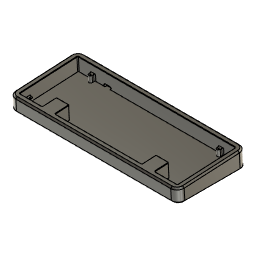
Vault 35 WKL MFR2 (Autodesk Fusion 360 design; units mm, degrees)
Autodesk Fusion 360 part; units mm, degrees
sketch "Outline Sketch" plane through (0, 0, 0) normal (0, 0, 1) x (1, 0, 0)
  line L0 (12.0219, -2.3777) -> (12.0219, 74.0723) construction
  line L1 (12.0219, 74.0723) -> (221.8219, 74.0723) construction
  line L2 (221.8219, 74.0723) -> (221.8219, -2.3777) construction
  line L3 (221.8219, -2.3777) -> (192.9969, -2.3777) construction
  line L4 (192.9969, -2.3777) -> (192.9969, 16.6723) construction
  line L5 (192.9969, 16.6723) -> (174.1969, 16.6723) construction
  line L6 (174.1969, 16.6723) -> (174.1969, -2.3777) construction
  line L7 (174.1969, -2.3777) -> (59.6469, -2.3777) construction
  line L8 (59.6469, -2.3777) -> (59.6469, 16.6723) construction
  line L9 (59.6469, 16.6723) -> (40.8469, 16.6723) construction
  line L10 (40.8469, 16.6723) -> (40.8469, -2.3777) construction
  line L11 (40.8469, -2.3777) -> (12.0219, -2.3777) construction
  line L12 (222.5719, -3.1277) -> (192.2469, -3.1277)
  line L13 (192.2469, -3.1277) -> (192.2469, 15.9223)
  line L14 (192.2469, 15.9223) -> (174.9469, 15.9223)
  line L15 (174.9469, 15.9223) -> (174.9469, -3.1277)
  line L16 (174.9469, -3.1277) -> (58.8969, -3.1277)
  line L17 (58.8969, -3.1277) -> (58.8969, 15.9223)
  line L18 (58.8969, 15.9223) -> (41.5969, 15.9223)
  line L19 (41.5969, 15.9223) -> (41.5969, -3.1277)
  line L20 (41.5969, -3.1277) -> (11.2719, -3.1277)
  line L21 (11.2719, -3.1277) -> (11.2719, 74.8223)
  line L22 (11.2719, 74.8223) -> (222.5719, 74.8223)
  line L23 (222.5719, 74.8223) -> (222.5719, -3.1277)
  line L24 (229.5719, -10.1277) -> (185.2469, -10.1277)
  line L25 (185.2469, -10.1277) -> (185.2469, 8.9223)
  line L26 (185.2469, 8.9223) -> (181.9469, 8.9223)
  line L27 (181.9469, 8.9223) -> (181.9469, -10.1277)
  line L28 (181.9469, -10.1277) -> (51.8969, -10.1277)
  line L29 (51.8969, -10.1277) -> (51.8969, 8.9223)
  line L30 (51.8969, 8.9223) -> (48.5969, 8.9223)
  line L31 (48.5969, 8.9223) -> (48.5969, -10.1277)
  line L32 (48.5969, -10.1277) -> (4.2719, -10.1277)
  line L33 (4.2719, -10.1277) -> (4.2719, 81.8223)
  line L34 (4.2719, 81.8223) -> (229.5719, 81.8223)
  line L35 (229.5719, 81.8223) -> (229.5719, -10.1277)
  line L36 (48.5969, -10.1277) -> (51.8969, -10.1277)
  line L37 (181.9469, -10.1277) -> (185.2469, -10.1277)
  dimension "d1" = 209.8
  dimension "d2" = 76.45
  dimension "d3" = 28.825
  dimension "d4" = 28.825
  dimension "d6" = 18.8
  dimension "d7" = 18.8
  dimension "d9" = 19.05
  dimension "d10" = 19.05
  dimension "d11" = 19.05
  dimension "d12" = 76.45
  dimension "d13" = 114.55
  dimension "d14" = -0.75
  dimension "d15" = -7.75
  constraint vertical L0
  constraint perpendicular L0 L1
  constraint perpendicular L1 L2
  constraint perpendicular L2 L3
  constraint perpendicular L3 L4
  constraint perpendicular L4 L5
  constraint perpendicular L5 L6
  constraint perpendicular L6 L7
  constraint perpendicular L7 L8
  constraint perpendicular L8 L9
  constraint perpendicular L9 L10
  constraint perpendicular L0 L11
  measures "d1" distance of L0 L2
  measures "d2" distance of L0.start L0.end
  measures "d3" distance of L0.start L10.end
  measures "d4" distance of L2.end L3.end
  measures "d6" distance of L8 L10
  measures "d7" distance of L4 L6
  measures "d9" distance of L9 L11
  measures "d10" distance of L3 L5
  measures "d11" distance of L7 L9
  measures "d12" distance of L1.end L2.end
  measures "d13" distance of L6 L8
extrude "Extrude1" add sketch "Outline Sketch" along normal blind 18.06
sketch "Angle Sketch" plane through (229.5719, 0, 0) normal (1, 0, 0) x (0, 1, 0)
  line L0 (-10.1277, 0) -> (81.8223, 0)
  line L1 (81.8223, 0) -> (81.8223, 18.06)
  line L2 (81.8223, 18.06) -> (-10.1277, 18.06)
  line L3 (-10.1277, 18.06) -> (-10.1277, 0)
  line L4 (-10.1277, 18.06) -> (-10.1277, -0.215)
  line L5 (-10.1277, -0.215) -> (89.7352, -5.4486)
  line L6 (-10.1277, -0.215) -> (89.8723, -0.215) construction
  dimension "d18" = 18.275
  dimension "d19" = 100
  dimension "d20" = 3
  constraint coincident L2.end L3.start
  constraint perpendicular L0 L4
  constraint horizontal L6
  measures "d18" distance of L2.end L4.end
  measures "d19" distance of L4.end L5.end
  measures "d20" angle of L5 L6
ref_plane "WorkPlane1" through (229.5719, 39.8037, -2.8318) normal (0, -0.052336, -0.99863) x (0, 0.99863, -0.052336)
sketch "Bottom Sketch for Angle" plane through (0, 0, 0) normal (0, 0, -1) x (1, 0, 0)
  line L0 (222.5719, -74.8223) -> (11.2719, -74.8223)
  line L1 (11.2719, -74.8223) -> (11.2719, 3.1277)
  line L2 (11.2719, 3.1277) -> (41.5969, 3.1277)
  line L3 (41.5969, 3.1277) -> (41.5969, -15.9223)
  line L4 (41.5969, -15.9223) -> (58.8969, -15.9223)
  line L5 (58.8969, -15.9223) -> (58.8969, 3.1277)
  line L6 (58.8969, 3.1277) -> (174.9469, 3.1277)
  line L7 (174.9469, 3.1277) -> (174.9469, -15.9223)
  line L8 (174.9469, -15.9223) -> (192.2469, -15.9223)
  line L9 (192.2469, -15.9223) -> (192.2469, 3.1277)
  line L10 (192.2469, 3.1277) -> (222.5719, 3.1277)
  line L11 (222.5719, 3.1277) -> (222.5719, -74.8223)
  line L12 (229.5719, 10.1277) -> (4.2719, 10.1277)
  line L13 (4.2719, 10.1277) -> (4.2719, -81.8223)
  line L14 (4.2719, -81.8223) -> (229.5719, -81.8223)
  line L15 (229.5719, -81.8223) -> (229.5719, 10.1277)
  line L16 (229.5719, -81.8223) -> (4.2719, -81.8223)
  line L17 (4.2719, -81.8223) -> (4.2719, 10.1277)
  line L18 (4.2719, 10.1277) -> (229.5719, 10.1277)
  line L19 (229.5719, 10.1277) -> (229.5719, -81.8223)
  constraint horizontal L16
  constraint vertical L17
  constraint horizontal L18
  constraint vertical L19
  constraint coincident L12.end L13.start
  constraint coincident L14.end L15.start
extrude "Extrude2" add sketch "Bottom Sketch for Angle" along normal up to surface contours L0 L1 L2 L3 L4 L5 L6 L7 L8 L9 L10 L11 | L12 L13 L14 L15 L16 L17 L18 L19 end surface through (229.5719, 39.8037, -2.8318) normal (0, -0.052336, -0.99863) offset 0
sketch "USB C Hole Internal Sketch" plane through (0, 74.8223, 0) normal (0, -1, 0) x (1, 0, 0)
  line L0 (11.2719, 0) -> (222.5719, 0)
  line L1 (222.5719, 0) -> (222.5719, 18.06)
  line L2 (222.5719, 18.06) -> (11.2719, 18.06)
  line L3 (11.2719, 18.06) -> (11.2719, 0)
  line L4 (11.2719, 0) -> (50.2469, 0) construction
  line L5 (50.2469, 0) -> (50.2469, 1.83) construction
  line L6 (54.9719, 3.66) -> (45.5219, 3.66)
  line L7 (45.5219, 3.66) -> (45.5219, 0)
  line L8 (45.5219, 0) -> (54.9719, 0)
  line L9 (54.9719, 0) -> (54.9719, 3.66)
  line L10 (54.9719, 3.66) -> (45.5219, 0) construction
  line L11 (45.5219, 3.66) -> (54.9719, 0) construction
  point P0 (50.2469, 1.83)
  dimension "d62" = 38.975
  dimension "d63" = 1.83
  dimension "d64" = 9.45
  dimension "d65" = 3.66
  constraint coincident L0.start L3.end
  constraint perpendicular L3 L4
  constraint perpendicular L4 L5
  constraint horizontal L6
  constraint perpendicular L6 L7
  constraint parallel L6 L8
  constraint parallel L7 L9
  constraint coincident L10 P0
  constraint coincident L11 P0
  constraint coincident P0 L5.end
  measures "d62" distance of L0.start L4.end
  measures "d63" distance of L4.end P0
  measures "d64" distance of L7.end L8.end
  measures "d65" distance of L6.end L7.end
extrude "Extrude5" cut sketch "USB C Hole Internal Sketch" against normal through all contours L0 L6 L7 L8 L9
fillet "Fillet3" radius 1.55 4 edges at (45.5219, 78.3223, 0) (54.9719, 78.3223, 0) (54.9719, 78.3223, 3.66) (45.5219, 78.3223, 3.66)
sketch "USB C Hole External Sketch" plane through (0, 81.8223, 0) normal (0, 1, 0) x (-1, 0, 0)
  line L0 (-47.0719, 0) -> (-53.4219, 0)
  arc A0 (-54.9719, 1.55) -> (-53.4219, 0) centre (-53.4219, 1.55) ccw
  line L1 (-54.9719, 1.55) -> (-54.9719, 2.11)
  arc A1 (-53.4219, 3.66) -> (-54.9719, 2.11) centre (-53.4219, 2.11) ccw
  line L2 (-53.4219, 3.66) -> (-47.0719, 3.66)
  arc A2 (-45.5219, 2.11) -> (-47.0719, 3.66) centre (-47.0719, 2.11) ccw
  line L3 (-45.5219, 2.11) -> (-45.5219, 1.55)
  arc A3 (-47.0719, 0) -> (-45.5219, 1.55) centre (-47.0719, 1.55) ccw
  line L4 (-4.2719, -5.0339) -> (-4.2719, 18.06)
  line L5 (-4.2719, 18.06) -> (-229.5719, 18.06)
  line L6 (-229.5719, 18.06) -> (-229.5719, -5.0339)
  line L7 (-229.5719, -5.0339) -> (-4.2719, -5.0339)
  line L8 (-43.2719, 5.91) -> (-57.2219, 5.91)
  line L9 (-57.2219, 5.91) -> (-57.2219, -2.25)
  line L10 (-57.2219, -2.25) -> (-43.2719, -2.25)
  line L11 (-43.2719, -2.25) -> (-43.2719, 5.91)
  line L12 (-43.2719, 5.91) -> (-57.2219, -2.25) construction
  line L13 (-57.2219, 5.91) -> (-43.2719, -2.25) construction
  point P0 (-50.2469, 1.83)
  point P1 (-50.2469, 1.83)
  dimension "d69" = 13.95
  dimension "d70" = 8.16
  dimension "d71" = 4.08
  dimension "d72" = 6.975
  constraint horizontal L8
  constraint perpendicular L8 L9
  constraint parallel L8 L10
  constraint parallel L9 L11
  constraint coincident L12 P1
  constraint coincident L13 P1
  measures "d69" distance of L9.end L10.end
  measures "d70" distance of L8.end L9.end
  measures "d71" distance of L8 P1
  measures "d72" distance of L9 P1
extrude "Extrude6" cut sketch "USB C Hole External Sketch" against normal blind 4.549 contours L8 L9 L10 L11
fillet "Fillet4" radius 3.8 4 edges at (57.2219, 79.5478, -2.25) (57.2219, 79.5478, 5.91) (43.2719, 79.5478, -2.25) (43.2719, 79.5478, 5.91)
chamfer "Chamfer3" distance 0.25 angle 45 8 edges at (56.1089, 81.8223, 4.797) (57.2219, 81.8223, 1.83) (56.1089, 81.8223, -1.137) (50.2469, 81.8223, -2.25) (44.3849, 81.8223, -1.137) (43.2719, 81.8223, 1.83) (44.3849, 81.8223, 4.797) (50.2469, 81.8223, 5.91)
fillet "Fillet1" radius 9 4 edges at (4.2719, -10.1277, 8.9225) (229.5719, -10.1277, 8.9225) (229.5719, 81.8223, 6.5131) (4.2719, 81.8223, 6.5131)
fillet "Fillet2" radius 1 12 edges at (58.8969, -3.1277, 9.03) (58.8969, 15.9223, 9.03) (41.5969, 15.9223, 9.03) (41.5969, -3.1277, 9.03) (174.9469, -3.1277, 9.03) (174.9469, 15.9223, 9.03) (192.2469, 15.9223, 9.03) (222.5719, -3.1277, 9.03) (192.2469, -3.1277, 9.03) (11.2719, -3.1277, 9.03) (11.2719, 74.8223, 9.03) (222.5719, 74.8223, 9.03)
chamfer "Chamfer1" distance 0.5 angle 45 24 edges at (116.9219, 74.8223, 18.06) (222.279, 74.5294, 18.06) (222.5719, 35.8473, 18.06) (222.279, -2.8348, 18.06) (207.4094, -3.1277, 18.06) (192.5398, -2.8348, 18.06) (192.2469, 6.3973, 18.06) (191.954, 15.6294, 18.06) (183.5969, 15.9223, 18.06) (175.2398, 15.6294, 18.06) (174.9469, 6.3973, 18.06) (174.654, -2.8348, 18.06) (116.9219, -3.1277, 18.06) (59.1898, -2.8348, 18.06) (58.8969, 6.3973, 18.06) (58.604, 15.6294, 18.06) (50.2469, 15.9223, 18.06) (41.8898, 15.6294, 18.06) (41.5969, 6.3973, 18.06) (41.304, -2.8348, 18.06) (26.4344, -3.1277, 18.06) (11.5648, -2.8348, 18.06) (11.2719, 35.8473, 18.06) (11.5648, 74.5294, 18.06)
chamfer "Chamfer2" distance 2 angle 45 16 edges at (116.9219, -10.1277, 18.06) (226.9359, -7.4917, 18.06) (229.5719, 35.8473, 18.06) (226.9359, 79.1862, 18.06) (116.9219, 81.8223, 18.06) (6.908, 79.1862, 18.06) (4.2719, 35.8473, 18.06) (6.908, -7.4917, 18.06) (116.9219, -10.1277, -0.215) (226.9359, -7.4917, -0.3531) (229.5719, 35.8473, -2.6244) (226.9359, 79.1862, -4.8957) (116.9219, 81.8223, -5.0339) (6.908, 79.1862, -4.8957) (4.2719, 35.8473, -2.6244) (6.908, -7.4917, -0.3531)
sketch "Screw Post Sketch" plane through (0, 0, 0) normal (0, 0, 1) x (-1, 0, 0)
  arc A0 (-222.5719, -73.8223) -> (-221.5719, -74.8223) centre (-221.5719, -73.8223) ccw
  line L0 (-221.5719, -74.8223) -> (-53.4219, -74.8223)
  arc A1 (-12.2719, -74.8223) -> (-11.2719, -73.8223) centre (-12.2719, -73.8223) ccw
  line L1 (-11.2719, -73.8223) -> (-11.2719, 2.1277)
  arc A2 (-11.2719, 2.1277) -> (-12.2719, 3.1277) centre (-12.2719, 2.1277) ccw
  line L2 (-12.2719, 3.1277) -> (-40.5969, 3.1277)
  arc A3 (-40.5969, 3.1277) -> (-41.5969, 2.1277) centre (-40.5969, 2.1277) ccw
  line L3 (-41.5969, 2.1277) -> (-41.5969, -14.9223)
  arc A4 (-42.5969, -15.9223) -> (-41.5969, -14.9223) centre (-42.5969, -14.9223) ccw
  line L4 (-42.5969, -15.9223) -> (-57.8969, -15.9223)
  arc A5 (-58.8969, -14.9223) -> (-57.8969, -15.9223) centre (-57.8969, -14.9223) ccw
  line L5 (-58.8969, -14.9223) -> (-58.8969, 2.1277)
  arc A6 (-58.8969, 2.1277) -> (-59.8969, 3.1277) centre (-59.8969, 2.1277) ccw
  line L6 (-59.8969, 3.1277) -> (-173.9469, 3.1277)
  arc A7 (-173.9469, 3.1277) -> (-174.9469, 2.1277) centre (-173.9469, 2.1277) ccw
  line L7 (-174.9469, 2.1277) -> (-174.9469, -14.9223)
  arc A8 (-175.9469, -15.9223) -> (-174.9469, -14.9223) centre (-175.9469, -14.9223) ccw
  line L8 (-175.9469, -15.9223) -> (-191.2469, -15.9223)
  arc A9 (-192.2469, -14.9223) -> (-191.2469, -15.9223) centre (-191.2469, -14.9223) ccw
  line L9 (-192.2469, -14.9223) -> (-192.2469, 2.1277)
  arc A10 (-192.2469, 2.1277) -> (-193.2469, 3.1277) centre (-193.2469, 2.1277) ccw
  line L10 (-193.2469, 3.1277) -> (-221.5719, 3.1277)
  arc A11 (-221.5719, 3.1277) -> (-222.5719, 2.1277) centre (-221.5719, 2.1277) ccw
  line L11 (-222.5719, 2.1277) -> (-222.5719, -73.8223)
  circle A12 centre (-31.1969, -71.4223) radius 2.25
  line L12 (-33.4469, -71.4223) -> (-33.4469, -73.6723)
  line L13 (-28.9469, -71.4223) -> (-28.9469, -73.6723)
  circle A13 centre (-202.6469, -71.4223) radius 2.25
  line L14 (-204.8969, -71.4223) -> (-204.8969, -73.6723)
  line L15 (-200.3969, -71.4223) -> (-200.3969, -73.6723)
  circle A14 centre (-14.4129, -7.5633) radius 2.25
  line L16 (-14.4129, -5.3133) -> (-12.4219, -5.3133)
  circle A15 centre (-219.4309, -7.5633) radius 2.25
  line L17 (-219.4309, -9.8133) -> (-221.4219, -9.8133)
  line L18 (-219.4309, -5.3133) -> (-221.4219, -5.3133)
  line L19 (-53.4219, -74.8223) -> (-53.4219, -77.2733)
  line L20 (-53.4219, -77.2733) -> (-47.0719, -77.2733)
  line L21 (-47.0719, -77.2733) -> (-47.0719, -74.8223)
  line L22 (-47.0719, -74.8223) -> (-12.2719, -74.8223)
  circle A16 centre (-77.9625, 1.9777) radius 1.15
  circle A17 centre (-155.8813, 1.9777) radius 1.15
  arc A18 (-75.6625, 3.1277) -> (-76.8125, 1.9777) centre (-75.6625, 1.9777) ccw
  arc A19 (-79.1125, 1.9777) -> (-80.2625, 3.1277) centre (-80.2625, 1.9777) ccw
  line L23 (-75.6625, 3.1277) -> (-80.2625, 3.1277)
  arc A20 (-157.0313, 1.9777) -> (-158.1813, 3.1277) centre (-158.1813, 1.9777) ccw
  arc A21 (-153.5813, 3.1277) -> (-154.7313, 1.9777) centre (-153.5813, 1.9777) ccw
  line L24 (-158.1813, 3.1277) -> (-153.5813, 3.1277)
  arc A22 (-28.9469, -73.6723) -> (-27.7969, -74.8223) centre (-27.7969, -73.6723) ccw
  arc A23 (-34.5969, -74.8223) -> (-33.4469, -73.6723) centre (-34.5969, -73.6723) ccw
  line L25 (-14.4129, -9.8133) -> (-12.4219, -9.8133)
  line L26 (-11.2719, -10.9633) -> (-11.2719, -13.8133)
  arc A24 (-11.2719, -10.9633) -> (-12.4219, -9.8133) centre (-12.4219, -10.9633) ccw
  line L27 (-11.2719, -4.1633) -> (-11.2719, -1.3133)
  arc A25 (-12.4219, -5.3133) -> (-11.2719, -4.1633) centre (-12.4219, -4.1633) ccw
  line L28 (-222.5719, -4.1633) -> (-222.5719, -1.3133)
  line L29 (-222.5719, -10.9633) -> (-222.5719, -13.8133)
  arc A26 (-221.4219, -9.8133) -> (-222.5719, -10.9633) centre (-221.4219, -10.9633) ccw
  arc A27 (-222.5719, -4.1633) -> (-221.4219, -5.3133) centre (-221.4219, -4.1633) ccw
  arc A28 (-200.3969, -73.6723) -> (-199.2469, -74.8223) centre (-199.2469, -73.6723) ccw
  arc A29 (-206.0469, -74.8223) -> (-204.8969, -73.6723) centre (-206.0469, -73.6723) ccw
  line L30 (-27.7969, -74.8223) -> (-34.5969, -74.8223)
  line L31 (-199.2469, -74.8223) -> (-206.0469, -74.8223)
  line L32 (-222.5719, -10.9633) -> (-222.5719, -4.1633)
  line L33 (-11.2719, -10.9633) -> (-11.2719, -4.1633)
  point P0 (-33.4469, -74.8223)
  point P1 (-28.9469, -74.8223)
  point P2 (-204.8969, -74.8223)
  point P3 (-200.3969, -74.8223)
  point P4 (-11.2719, -5.3133)
  point P5 (-222.5719, -9.8133)
  point P6 (-222.5719, -5.3133)
  point P7 (-76.8125, 3.1277)
  point P8 (-79.1125, 3.1277)
  point P9 (-154.7313, 3.1277)
  point P10 (-157.0313, 3.1277)
  point P11 (-11.2719, -9.8133)
  dimension "d33" = 4.5
  dimension "d34" = 3.4
  dimension "d35" = 19.925
  dimension "d36" = 4.5
  dimension "d37" = 19.925
  dimension "d38" = 3.4
  dimension "d39" = 4.5
  dimension "d40" = 10.691
  dimension "d41" = 3.141
  dimension "d42" = 4.5
  dimension "d43" = 10.691
  dimension "d44" = 3.141
  dimension "d80" = 2.3
  dimension "d81" = 2.3
  dimension "d84" = 1.15
  dimension "d85" = 1.15
  dimension "d94" = 116.05
  dimension "d95" = 19.0656
  dimension "d96" = 19.0656
  dimension "d108" = 1.15
  dimension "d110" = 1.15
  dimension "d113" = 1.15
  dimension "d114" = 1.15
  dimension "d117" = 1.15
  dimension "d118" = 1.15
  dimension "d119" = 4
  dimension "d120" = 1.15
  dimension "d121" = 4
  dimension "d122" = 1.15
  dimension "d123" = 4
  dimension "d124" = 4
  dimension "d125" = 1.15
  dimension "d126" = 1.15
  dimension "d129" = 1.15
  dimension "d130" = 1.15
  constraint coincident A12 L12.start
  constraint coincident L0 P0
  constraint tangent A12 L12
  constraint perpendicular L0 L12
  constraint coincident A12 L13.start
  constraint coincident L0 P1
  constraint tangent A12 L13
  constraint perpendicular L0 L13
  constraint coincident A13 L14.start
  constraint coincident L0 P2
  constraint tangent A13 L14
  constraint perpendicular L0 L14
  constraint coincident A13 L15.start
  constraint tangent A13 L15
  constraint perpendicular L0 L15
  constraint coincident A14 L16.start
  constraint coincident L1 P4
  constraint tangent A14 L16
  constraint perpendicular L1 L16
  constraint coincident A15 L17.start
  constraint coincident L11 P5
  constraint tangent A15 L17
  constraint perpendicular L11 L17
  constraint coincident A15 L18.start
  constraint coincident L11 P6
  constraint tangent A15 L18
  constraint perpendicular L11 L18
  constraint coincident L6 P8
  constraint tangent A19 L23
  constraint coincident L6 P9
  constraint coincident L6 P10
  constraint tangent A21 L24
  constraint coincident P1 L13
  constraint tangent L13 A22
  constraint coincident P0 L12
  constraint tangent L12 A23
  constraint horizontal L25
  constraint coincident A14 L25.start
  constraint coincident L1 P11
  constraint tangent A14 L25
  constraint perpendicular L25 L26
  constraint coincident P11 L26
  constraint coincident P11 L25
  constraint tangent L26 A24
  constraint tangent L25 A24
  constraint perpendicular L16 L27
  constraint coincident P4 L27
  constraint coincident P4 L16
  constraint tangent L27 A25
  constraint tangent L16 A25
  constraint perpendicular L18 L28
  constraint perpendicular L17 L29
  constraint coincident P5 L17
  constraint coincident P5 L29
  constraint tangent L17 A26
  constraint tangent L29 A26
  constraint coincident P6 L18
  constraint coincident P6 L28
  constraint tangent L18 A27
  constraint tangent L28 A27
  constraint coincident P3 L15
  constraint tangent L15 A28
  constraint coincident P2 L14
  constraint tangent L14 A29
  constraint tangent A23 L30
  constraint tangent A29 L31
  measures "d33" diameter of A12
  measures "d34" distance of L0 A12.centre
  measures "d35" distance of L1 A12.centre
  measures "d36" diameter of A13
  measures "d37" distance of L11 A13.centre
  measures "d38" distance of L0 A13.centre
  measures "d39" diameter of A14
  measures "d40" distance of L2 A14.centre
  measures "d41" distance of L1 A14.centre
  measures "d42" diameter of A15
  measures "d43" distance of L10 A15.centre
  measures "d44" distance of L11 A15.centre
  measures "d80" diameter of A16
  measures "d81" diameter of A17
  measures "d84" distance of L6 A16.centre
  measures "d85" distance of L6 A17.centre
  measures "d94" distance of L5 L7
  measures "d95" distance of L5 A16.centre
  measures "d96" distance of L7 A17.centre
  measures "d108" radius of A18
  measures "d110" radius of A19
  measures "d113" radius of A20
  measures "d114" radius of A21
  measures "d117" radius of A22
  measures "d118" radius of A23
  measures "d119" distance of P11 L26.end
  measures "d120" radius of A24
  measures "d121" distance of P4 L27.end
  measures "d122" radius of A25
  measures "d123" distance of P6 L28.end
  measures "d124" distance of P5 L29.end
  measures "d125" radius of A26
  measures "d126" radius of A27
  measures "d129" radius of A28
  measures "d130" radius of A29
extrude "Extrude4" add sketch "Screw Post Sketch" along normal blind 8.41 contours L0 A13 L14 L15 A28 A29 L31 | L11 A15 L17 L18 A26 A27 L32 | A13 | A15 | A12 L12 L13 L22 A22 A23 L30 | A12 | L1 A14 L16 L25 A24 A25 L33 | A14 | L6 A17 A20 L24 | L6 A17 A21 L24 | A17 | L6 A16 A19 L23 | L6 A16 A18 L23 | A16
hole "Hole2" at (31.1969, 71.4223, 8.41) direction (0, 0, -1) diameter 1.8 depth 4 tip angle 180
hole "Hole3" at (202.6469, 71.4223, 8.41) direction (0, 0, -1) diameter 1.8 depth 4 tip angle 180
hole "Hole4" at (219.4309, 7.5633, 8.41) direction (0, 0, -1) diameter 1.8 depth 4 tip angle 180
hole "Hole5" at (14.4129, 7.5633, 8.41) direction (0, 0, -1) diameter 1.8 depth 4 tip angle 180
extrude "Extrude3" add 1 faces at (82.3719, 21.188, -1.8562) along direction (0, 0.052336, 0.99863) blind 1
move_body "Move1" bodies 1 to x (1, 0, 0) y (0, 0.99863, 0.052336) z (0, -0.052336, 0.99863) at (0, 0.0795, 0.5325)
equation "d45 = 7.9 mm + 0.51 mm"
equation "d62 = 0.875 mm + 2 * 19.05 mm"
equation "d63 = ( 3.66 / 2 ) * 1 mm"
equation "d64 = ( 4.725 * 2 ) * 1 mm"
equation "d71 = d70 / 2"
equation "d72 = d69 / 2"
equation "d73 = -3.5 mm - 1.049 mm"
equation "d84 = d80 / 2"
equation "d85 = d81 / 2"
equation "d95 = 1.5 mm + 17.565625 mm"
equation "d96 = d95"
equation "d108 = ( 2.3 / 2 ) * 1 mm"
equation "d110 = ( 2.3 / 2 ) * 1 mm"
equation "d113 = ( 2.3 / 2 ) * 1 mm"
equation "d114 = ( 2.3 / 2 ) * 1 mm"
